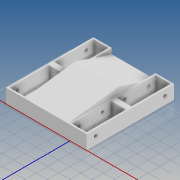
# Autodesk Inventor part: prototype 1
Saved by Autodesk Inventor 2020 (Build 240168000, 168)
## iProperties
Created: 2019-12-03
Part Number: prototype 1
Material: Generic
Document SubType Name: Modeling
Designer: Berkant
Density: 1 g/cm^3
Appearance: Default
Author: Berkant
Autodesk Inventor part; units mm, degrees
ref_plane "YZ Plane" through (0, 0, 0) normal (1, 0, 0) x (0, 1, 0)
ref_plane "XZ Plane" through (0, 0, 0) normal (0, 1, 0) x (-1, 0, 0)
ref_plane "XY Plane" through (0, 0, 0) normal (0, 0, 1) x (1, 0, 0)
sketch "Sketch1" plane through (0, 0, 0) normal (0, 1, 0) x (-1, 0, 0)
  line L0 (0, 0) -> (84, 0)
  line L1 (84, 0) -> (84, -156)
  line L2 (84, -156) -> (0, -156)
  line L3 (0, -156) -> (0, 0)
  line L4 (84, 0) -> (84, -3)
  line L5 (84, -3) -> (81, -3) construction
  line L6 (0, -156) -> (0, -153)
  line L7 (0, -153) -> (3, -153) construction
  line L8 (81, -3) -> (3, -3)
  line L9 (3, -3) -> (3, -153)
  line L10 (3, -153) -> (81, -153)
  line L11 (81, -153) -> (81, -3)
  dimension "d0" = 84
  dimension "d1" = 156
  dimension "d2" = 3
  dimension "d3" = 3
  dimension "d4" = 3
  dimension "d5" = 3
  constraints: 24 end point, 4 parallel, 4 perpendicular, 2 horizontal, 2 point on line
  measures "d0" distance of L1.end L2.end
  measures "d1" distance of L0.end L1.end
  measures "d2" distance of L0.end L4.end
  measures "d3" distance of L4.end L5.end
  measures "d4" distance of L2.end L6.end
  measures "d5" distance of L6.end L7.end
extrude "Extrusion1" add sketch "Sketch1" along normal blind 15 contours L0 L1 L2 L3 | L11 L10 L9 L8
sketch "Sketch2" plane through (0, 15, 0) normal (0, 1, 0) x (1, 0, 0)
  line L0 (-84, 156) -> (-84, 0) projected
  line L1 (-84, 0) -> (-84, 3)
  line L2 (-84, 3) -> (-81, 3) construction
  line L3 (0, 0) -> (0, 156) projected
  line L4 (0, 156) -> (0, 153)
  line L5 (0, 153) -> (-3, 153) construction
  line L6 (-81, 3) -> (-3, 3)
  line L7 (-3, 3) -> (-3, 153)
  line L8 (-3, 153) -> (-81, 153)
  line L9 (-81, 153) -> (-81, 3)
  dimension "d8" = 3
  dimension "d9" = 3
  dimension "d10" = 3
  dimension "d11" = 3
  constraints: 16 end point, 3 perpendicular, 2 parallel, 2 point on line, 1 horizontal
  measures "d8" distance of L0.end L1.end
  measures "d9" distance of L1.end L2.end
  measures "d10" distance of L3.end L4.end
  measures "d11" distance of L4.end L5.end
extrude "Extrusion2" cut sketch "Sketch2" against normal blind 12
sketch "Sketch5" plane through (0, 0, 0) normal (1, 0, 0) x (0, 0, -1)
  line L0 (0, 15) -> (156, 15) projected
  line L1 (0, 15) -> (0, 0)
  line L2 (156, 0) -> (0, 0) projected
  line L3 (0, 0) -> (156, 0)
  line L4 (156, 0) -> (156, 15)
  line L5 (156, 15) -> (153, 15)
  line L6 (3, 3) -> (153, 3) projected
  line L7 (153, 15) -> (153, 3)
  line L8 (153, 3) -> (83, 3)
  line L9 (83, 3) -> (83, 15)
  line L10 (0, 15) -> (3, 15)
  line L11 (3, 15) -> (3, 3) projected
  line L12 (3, 15) -> (3, 3)
  line L13 (3, 3) -> (73, 3)
  line L14 (73, 3) -> (73, 15)
  line L15 (83, 15) -> (73, 15)
  dimension "d18" = 3
  dimension "d19" = 12
  dimension "d20" = 70
  dimension "d21" = 70
  constraints: 24 end point, 5 perpendicular, 5 point on line, 2 vertical
  measures "d18" distance of L4.end L5.end
  measures "d19" distance of L5.end L6.end
  measures "d20" distance of L6.end L8.end
  measures "d21" distance of L6.start L13.end
extrude "Extrusion3" add sketch "Sketch5" along normal blind 27 contours L0 L11 L6 L7 L4 L2 L1 | L0 L9 L6 L14
sketch "Sketch6" plane through (27, 0, 0) normal (1, 0, 0) x (0, 0, -1)
  line L0 (0, 15) -> (0, 0) projected
  line L1 (156, 0) -> (156, 15) projected
  line L2 (0, 0) -> (156, 0)
  line L3 (156, 0) -> (156, 15)
  line L4 (156, 15) -> (0, 15)
  line L5 (0, 15) -> (0, 0)
  constraints: 8 end point, 2 parallel, 1 horizontal, 1 perpendicular
extrude "Extrusion4" add sketch "Sketch6" along normal blind 3
sketch "Sketch8" plane through (-84, 0, -156) normal (-1, 0, 0) x (0, 0, 1)
  line L0 (3, 15) -> (3, 3) projected
  line L1 (3, 15) -> (3, 3)
  line L2 (3, 3) -> (73, 3)
  line L3 (73, 3) -> (73, 15)
  line L4 (156, 15) -> (153, 15)
  line L5 (153, 15) -> (153, 3)
  line L6 (153, 3) -> (83, 3)
  line L7 (83, 3) -> (83, 15)
  line L8 (83, 15) -> (73, 15)
  line L9 (156, 0) -> (156, 15) projected
  line L10 (156, 15) -> (156, 0)
  line L11 (156, 0) -> (0, 0)
  line L12 (0, 0) -> (0, 15) projected
  line L13 (0, 0) -> (0, 15)
  line L14 (0, 15) -> (3, 15)
  dimension "d35" = 70
  dimension "d38" = 12
  dimension "d39" = 70
  constraints: 24 end point, 6 perpendicular, 2 vertical
  measures "d35" distance of L0.end L2.end
  measures "d38" distance of L4.end L5.end
  measures "d39" distance of L5.end L6.end
extrude "Extrusion5" add sketch "Sketch8" along normal blind 27
sketch "Sketch9" plane through (-111, 0, -156) normal (-1, 0, 0) x (0, 0, 1)
  line L0 (0, 0) -> (156, 0) projected
  line L1 (156, 15) -> (156, 0) projected
  line L2 (0, 0) -> (156, 0)
  line L3 (156, 0) -> (156, 15)
  line L4 (156, 15) -> (0, 15)
  line L5 (0, 15) -> (0, 0)
  constraints: 8 end point, 2 parallel, 1 horizontal, 1 perpendicular
extrude "Extrusion6" add sketch "Sketch9" along normal blind 3
sketch "Sketch10" plane through (0, 15, 0) normal (0, 1, 0) x (1, 0, 0)
  line L0 (-3, 3) -> (-81, 3) projected
  line L1 (-3, 3) -> (-3, 0)
  line L2 (30, 0) -> (-114, 0) projected
  line L3 (30, 156) -> (30, 0) projected
  line L4 (30, 156) -> (-3, 156)
  line L5 (-3, 156) -> (-3, 0)
  line L6 (-3, 0) -> (30, 0)
  line L7 (30, 0) -> (30, 156)
  line L8 (-81, 3) -> (-81, 0)
  line L9 (-114, 156) -> (30, 156) projected
  line L10 (-114, 156) -> (-81, 156)
  line L11 (-81, 156) -> (-81, 0)
  line L12 (-81, 0) -> (-114, 0)
  line L13 (-114, 0) -> (-114, 156)
  line L14 (27, 153) -> (27, 83) projected
  line L15 (0, 83) -> (0, 153) projected
  line L16 (27, 153) -> (0, 153)
  line L17 (0, 153) -> (0, 83)
  line L18 (0, 83) -> (27, 83)
  line L19 (27, 83) -> (27, 153)
  line L20 (0, 73) -> (27, 73) projected
  line L21 (0, 3) -> (27, 3) projected
  line L22 (27, 73) -> (0, 73)
  line L23 (0, 73) -> (0, 3)
  line L24 (0, 3) -> (27, 3)
  line L25 (27, 3) -> (27, 73)
  line L26 (-84, 153) -> (-84, 83) projected
  line L27 (-84, 83) -> (-111, 83) projected
  line L28 (-84, 153) -> (-111, 153)
  line L29 (-111, 153) -> (-111, 83)
  line L30 (-111, 83) -> (-84, 83)
  line L31 (-84, 83) -> (-84, 153)
  line L32 (-84, 73) -> (-84, 3) projected
  line L33 (-84, 3) -> (-111, 3) projected
  line L34 (-84, 73) -> (-111, 73)
  line L35 (-111, 73) -> (-111, 3)
  line L36 (-111, 3) -> (-84, 3)
  line L37 (-84, 3) -> (-84, 73)
  point P0 (0, 0)
  constraints: 52 end point, 12 parallel, 7 perpendicular, 6 horizontal, 2 point on line, 1 vertical
extrude "Extrusion7" add sketch "Sketch10" along normal blind 10 contours L5 L4 L3 L2 L1 | L8 L2 L13 L9 L11
sketch "Sketch11" plane through (-114, 0, -156) normal (-1, 0, 0) x (0, 0, 1)
  line L0 (0, 25) -> (16, 25)
  line L1 (16, 25) -> (16, 13.8)
  circle A0 centre (16, 13.8) radius 3
  line L2 (156, 15) -> (156, 25) projected
  line L3 (156, 25) -> (140, 25)
  line L4 (140, 25) -> (140, 13.8)
  circle A1 centre (140, 13.8) radius 3
  dimension "d117" = 16
  dimension "d118" = 11.2
  dimension "d119" = 6
  dimension "d120" = 16
  dimension "d121" = 11.2
  dimension "d122" = 6
  constraints: 8 end point, 2 centre point, 2 coincident, 2 horizontal, 2 perpendicular
  measures "d117" distance of L0.start L0.end
  measures "d118" distance of L0.end L1.end
  measures "d119" diameter of A0
  measures "d120" distance of L2.end L3.end
  measures "d121" distance of L3.end L4.end
  measures "d122" diameter of A1
extrude "Extrusion8" cut sketch "Sketch11" against normal blind 32
sketch "Sketch12" plane through (30, 0, 0) normal (1, 0, 0) x (0, 0, -1)
  line L0 (0, 25) -> (16, 25)
  line L1 (0, 25) -> (16, 25) construction
  line L2 (16, 25) -> (16, 13.8)
  circle A0 centre (16, 13.8) radius 3
  line L3 (156, 25) -> (140, 25)
  line L4 (140, 25) -> (140, 13.8)
  circle A1 centre (140, 13.8) radius 3
  dimension "d98" = 16
  dimension "d99" = 0
  dimension "d100" = 11.2
  dimension "d101" = 6
  dimension "d102" = 16
  dimension "d103" = 11.2
  dimension "d104" = 6
  constraints: 10 end point, 2 centre point, 2 coincident, 2 horizontal, 2 perpendicular, 1 collinear
  measures "d98" distance of L0.start L0.end
  measures "d99" distance between parallel lines of L0 L1
  measures "d100" distance of L0.end L2.end
  measures "d101" diameter of A0
  measures "d102" distance of L3.start L3.end
  measures "d103" distance of L3.end L4.end
  measures "d104" diameter of A1
extrude "Extrusion9" cut sketch "Sketch12" against normal blind 32
sketch "Sketch13" plane through (0, 3, -3) normal (1, 0, 0) x (0, 0, -1)
  line L0 (0, 22) -> (70, 22) projected
  line L1 (0, 22) -> (55, 22)
  line L2 (55, 22) -> (54.9973, 12)
  circle A0 centre (54.9973, 12) radius 2.5
  line L3 (80, 22) -> (95, 22)
  line L4 (80, 22) -> (150, 22) projected
  line L5 (95, 22) -> (95, 12)
  circle A1 centre (95, 12) radius 2.5
  point P0 (-3, -3)
  dimension "d105" = 55
  dimension "d106" = 10
  dimension "d107" = 5
  dimension "d108" = 15
  dimension "d109" = 10
  dimension "d110" = 5
  constraints: 8 end point, 2 centre point, 2 coincident, 2 point on line, 1 perpendicular
  measures "d105" distance of L0.start L1.end
  measures "d106" distance of L1.end L2.end
  measures "d107" diameter of A0
  measures "d108" distance of L3.start L3.end
  measures "d109" distance of L3.end L5.end
  measures "d110" diameter of A1
sketch "Sketch14" plane through (-84, 3, -153) normal (-1, 0, 0) x (0, 0, 1)
  line L0 (70, 0) -> (70, 22) projected
  line L1 (70, 22) -> (55, 22)
  line L2 (55, 22) -> (55, 12)
  circle A0 centre (55, 12) radius 2.5
  line L3 (80, 22) -> (95, 22)
  line L4 (95, 22) -> (95, 12)
  circle A1 centre (95, 12) radius 2.5
  point P0 (153, -3)
  point P1 (0, 22)
  point P2 (150, 22)
  dimension "d111" = 15
  dimension "d112" = 10
  dimension "d113" = 5
  dimension "d114" = 15
  dimension "d115" = 10
  dimension "d116" = 5
  constraints: 8 end point, 2 centre point, 2 coincident, 2 perpendicular
  measures "d111" distance of L0.end L1.end
  measures "d112" distance of L1.end L2.end
  measures "d113" diameter of A0
  measures "d114" distance of L3.start L3.end
  measures "d115" distance of L3.end L4.end
  measures "d116" diameter of A1
extrude "Extrusion10" cut sketch "Sketch14" against normal blind 10
extrude "Extrusion11" cut sketch "Sketch13" against normal blind 10
sketch "Sketch15" plane through (-81, 3, -3) normal (1, 0, 0) x (0, 0, -1)
  line L0 (-3, 22) -> (87.2546, 33.7556)
  line L1 (87.2546, 33.7556) -> (153, 12)
  line L2 (-3, 22) -> (-3, 12)
  line L3 (153, 12) -> (150, 12)
  line L4 (153, 12) -> (-3, 12)
  constraints: 10 end point, 1 collinear
extrude "Extrusion12" add sketch "Sketch15" along normal up to surface (78 mm away)
body "Solid1"
